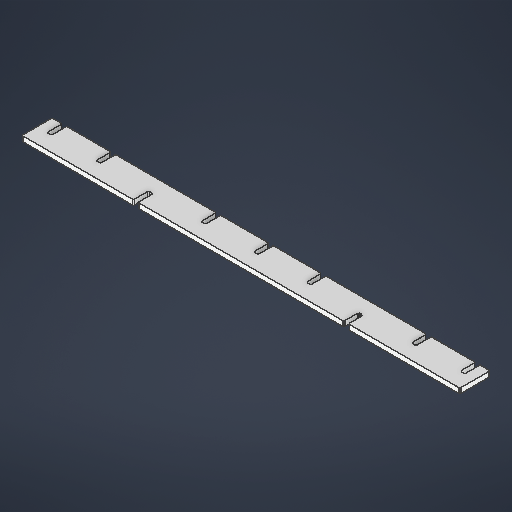
# Autodesk Inventor part: slats
Saved by Autodesk Inventor 2027.1 (Build 311270010, 270A)
## iProperties
Created: 2025-09-12
Part Number: slats
Material: Foam Core Board
Document SubType Name: Modeling
Designer: Nick
Density: 0.141998 g/cm^3
Appearance: Default(1)
Mass: 8.83359 g
Surface Area: 308 cm^2
Volume: 62.2093 cm^3
Author: Nick
Autodesk Inventor part; units mm, degrees
ref_plane "YZ Plane" through (0, 0, 0) normal (1, 0, 0) x (0, 1, 0)
ref_plane "XZ Plane" through (0, 0, 0) normal (0, 1, 0) x (-1, 0, 0)
ref_plane "XY Plane" through (0, 0, 0) normal (0, 0, 1) x (1, 0, 0)
sketch "Sketch1" plane through (0, 0, 0) normal (0, 1, 0) x (-1, 0, 0)
  line L0 (0, 0) -> (435, 0)
  line L1 (435, 0) -> (435, -30)
  line L2 (435, -30) -> (0, -30)
  line L3 (0, -30) -> (0, 0)
  dimension "d0" = 435
  dimension "d1" = 30
  constraints: 8 end point, 2 parallel, 1 horizontal, 1 perpendicular
  measures "d0" distance of L1.end L2.end
  measures "d1" distance of L0.end L1.end
extrude "Extrusion1" add sketch "Sketch1" along normal blind 5
sketch "Sketch2" plane through (0, 5, 0) normal (0, 1, 0) x (1, 0, 0)
  line L0 (0, 30) -> (-435, 30) projected
  line L1 (-435, 30) -> (-425, 30)
  line L2 (-425, 30) -> (-420.5, 30)
  line L3 (-420.5, 30) -> (-420.5, 15)
  line L4 (-420.5, 15) -> (-425, 15)
  line L5 (-425, 15) -> (-425, 30)
  line L6 (-420.5, 30) -> (-219.75, 30)
  line L7 (-219.75, 30) -> (-215.25, 30)
  line L8 (-215.25, 30) -> (-215.25, 15)
  line L9 (-215.25, 15) -> (-219.75, 15)
  line L10 (-219.75, 15) -> (-219.75, 30)
  line L11 (-215.25, 30) -> (-14.5, 30)
  line L12 (-14.5, 30) -> (-10, 30)
  line L13 (-10, 30) -> (-10, 15)
  line L14 (-10, 15) -> (-14.5, 15)
  line L15 (-14.5, 15) -> (-14.5, 30)
  point P0 (0, 0)
  dimension "d4" = 10
  dimension "d5" = 4.5
  dimension "d6" = 15
  dimension "d7" = 200.75
  dimension "d8" = 4.5
  dimension "d9" = 15
  dimension "d10" = 200.75
  dimension "d11" = 4.5
  dimension "d12" = 15
  constraints: 30 end point, 6 parallel, 3 horizontal, 3 perpendicular, 3 point on line
  measures "d4" distance of L0.end L1.end
  measures "d5" distance of L3.end L4.end
  measures "d6" distance of L2.end L3.end
  measures "d7" distance of L2.end L6.end
  measures "d8" distance of L8.end L9.end
  measures "d9" distance of L7.end L8.end
  measures "d10" distance of L7.end L11.end
  measures "d11" distance of L13.end L14.end
  measures "d12" distance of L12.end L13.end
extrude "Extrusion2" cut sketch "Sketch2" against normal blind 5
sketch "Sketch6" plane through (0, 5, 0) normal (0, 1, 0) x (1, 0, 0)
  line L0 (-14.5, 30) -> (-14.5, 15) projected
  line L1 (-14.5, 15) -> (-58.5, 15)
  line L2 (-14.5, 30) -> (-215.25, 30) projected
  line L3 (-58.5, 15) -> (-63, 15)
  line L4 (-63, 15) -> (-63, 30)
  line L5 (-63, 30) -> (-58.5, 30)
  line L6 (-58.5, 30) -> (-58.5, 15)
  line L7 (-63, 15) -> (-110.75, 15)
  line L8 (-110.75, 15) -> (-115.25, 15)
  line L9 (-115.25, 15) -> (-115.25, 30)
  line L10 (-115.25, 30) -> (-110.75, 30)
  line L11 (-110.75, 30) -> (-110.75, 15)
  line L12 (-115.25, 15) -> (-163, 15)
  line L13 (-163, 15) -> (-167.5, 15)
  line L14 (-167.5, 15) -> (-167.5, 30)
  line L15 (-167.5, 30) -> (-163, 30)
  line L16 (-163, 30) -> (-163, 15)
  line L17 (-435, 0) -> (0, 0) projected
  line L18 (-217.5, 0) -> (-217.5, 47.2454)
  line L19 (-376.5, 15) -> (-372, 15)
  line L20 (-372, 15) -> (-372, 30)
  line L21 (-372, 30) -> (-376.5, 30)
  line L22 (-376.5, 30) -> (-376.5, 15)
  line L23 (-372, 15) -> (-324.25, 15)
  line L24 (-324.25, 15) -> (-319.75, 15)
  line L25 (-319.75, 15) -> (-319.75, 30)
  line L26 (-319.75, 30) -> (-324.25, 30)
  line L27 (-324.25, 30) -> (-324.25, 15)
  line L28 (-319.75, 15) -> (-272, 15)
  line L29 (-272, 15) -> (-267.5, 15)
  line L30 (-267.5, 15) -> (-267.5, 30)
  line L31 (-267.5, 30) -> (-272, 30)
  line L32 (-272, 30) -> (-272, 15)
  line L33 (-110.75, 15) -> (-115.25, 15)
  line L34 (-115.25, 15) -> (-115.25, 0)
  line L35 (-115.25, 0) -> (-110.75, 0)
  line L36 (-110.75, 0) -> (-110.75, 15)
  line L37 (-319.75, 15) -> (-324.25, 15)
  line L38 (-324.25, 15) -> (-324.25, 0)
  line L39 (-324.25, 0) -> (-319.75, 0)
  line L40 (-319.75, 0) -> (-319.75, 15)
  dimension "d40" = 44
  dimension "d41" = 4.5
  dimension "d42" = 47.75
  dimension "d43" = 4.5
  dimension "d44" = 47.75
  dimension "d45" = 4.5
  dimension "d48" = 15
  dimension "d49" = 4.5
  dimension "d50" = 106.75
  constraints: 76 end point, 12 symmetric about line, 11 parallel, 7 horizontal, 6 point on line, 5 perpendicular, 1 midpoint, 1 vertical
  measures "d40" distance of L0.end L1.end
  measures "d41" distance of L4.end L5.end
  measures "d42" distance of L3.end L7.end
  measures "d43" distance of L9.end L10.end
  measures "d44" distance of L8.end L12.end
  measures "d45" distance of L14.end L15.end
  measures "d48" distance of L37.end L38.end
  measures "d49" distance of L24.start L24.end
  measures "d50" distance from line of L18 L38.end
extrude "Extrusion6" cut sketch "Sketch6" against normal blind 5 contours L19 L22 L21 L20 | L32 L31 L30 L29 | L17 L38 L24 L40 | L6 L3 L4 L2 | L36 L17 L34 L8 | L16 L13 L14 L2
fillet "Fillet2" radius 1 39 edges at (0, 2.5, -30) (-10, 2.5, -15) (-14.5, 2.5, -15) (-14.5, 2.5, -30) (0, 2.5, 0) (-110.75, 2.5, 0) (-115.25, 2.5, 0) (-115.25, 2.5, -15) (-110.75, 2.5, -15) (-63, 2.5, -15) (-58.5, 2.5, -15) (-58.5, 2.5, -30) (-63, 2.5, -30) (-163, 2.5, -15) (-167.5, 2.5, -15) (-163, 2.5, -30) (-167.5, 2.5, -30) (-219.75, 2.5, -30) (-215.25, 2.5, -30) (-215.25, 2.5, -15) (-219.75, 2.5, -15) (-267.5, 2.5, -15) (-272, 2.5, -15) (-272, 2.5, -30) (-267.5, 2.5, -30) (-319.75, 2.5, 0) (-324.25, 2.5, 0) (-324.25, 2.5, -15) (-319.75, 2.5, -15) (-376.5, 2.5, -30) (-376.5, 2.5, -15) (-372, 2.5, -15) (-372, 2.5, -30) (-420.5, 2.5, -30) (-425, 2.5, -30) (-420.5, 2.5, -15) (-425, 2.5, -15) (-435, 2.5, 0) (-435, 2.5, -30)
body "Solid1"
